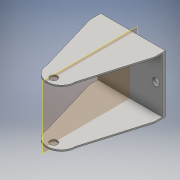
# Autodesk Inventor part: Thin Wheel Mount
Saved by Autodesk Inventor 2016 (Build 200138000, 138)
## iProperties
Created: 2016-05-08
Part Number: Thin Wheel Mount
Material: Generic
Document SubType Name: Modeling
Designer: Kenneth Daniel
Density: 1 g/cm^3
Appearance: Default
Author: Kenneth Daniel
Autodesk Inventor part; units mm, degrees
ref_plane "YZ Plane" through (0, 0, 0) normal (1, 0, 0) x (0, 1, 0)
ref_plane "XZ Plane" through (0, 0, 0) normal (0, 1, 0) x (-1, 0, 0)
ref_plane "XY Plane" through (0, 0, 0) normal (0, 0, 1) x (1, 0, 0)
sketch "Sketch1" plane through (0, 0, 0) normal (0, 0, 1) x (1, 0, 0)
  line L0 (-22.5, -30) -> (-22.5, 30)
  line L1 (-22.5, 30) -> (22.5, 30)
  line L2 (22.5, 30) -> (22.5, -30)
  line L3 (22.5, -30) -> (-22.5, -30)
  line L4 (-22.5, -30) -> (22.5, 30) construction
  line L5 (-22.5, 30) -> (22.5, -30) construction
  line L6 (-22.5, 30) -> (-22.5, 22.5)
  line L7 (0, -30) -> (0, -20)
  line L8 (0, -20) -> (-10, -20)
  line L9 (-10, -20) -> (10, -20)
  line L10 (-22.5, 22.5) -> (-10, -20)
  line L11 (22.5, 30) -> (22.5, 22.5)
  line L12 (22.5, 22.5) -> (10, -20)
  arc A0 (-10, -20) -> (10, -20) centre (0, -20) ccw
  point P0 (0, 0)
  dimension "d0" = 60
  dimension "d1" = 45
  dimension "d2" = 7.5
  dimension "d3" = 10
  dimension "d4" = 10
  dimension "d5" = 20
  dimension "d6" = 7.5
  constraints: 26 end point, 3 midpoint, 3 point on circle, 3 point on line, 2 parallel, 2 perpendicular, 2 vertical, 1 centre point
  measures "d0" distance of L0.start L0.end
  measures "d1" distance of L0.end L1.end
  measures "d2" distance of L0.end L6.end
  measures "d3" distance of L7.start L7.end
  measures "d4" distance of L7.end L8.end
  measures "d5" distance of L8.end L9.end
  measures "d6" distance of L1.end L11.end
extrude "Extrusion1" add sketch "Sketch1" along normal blind 40 contours L0 L1 L2 L12 L9 L8 L10 | A0 L8 L7 | L7 L9 A0
sketch "Sketch2" plane through (0, 0, 0) normal (1, 0, 0) x (0, 1, 0)
  line L0 (30, 0) -> (30, 40) projected
  line L1 (30, 40) -> (30, 0)
  line L2 (-20, 0) -> (-30, 0) projected
  line L3 (30, 0) -> (-30, 0)
  line L4 (-30, 0) -> (-30, 1)
  line L5 (-30, 0) -> (-30, 40) projected
  line L6 (30, 40) -> (-30, 40)
  line L7 (-30, 40) -> (-30, 39)
  line L8 (-30, 39) -> (27.8612, 39)
  line L9 (30, 40) -> (22.5, 40) projected
  line L10 (-30, 1) -> (27.8612, 1)
  line L11 (27.8612, 1) -> (27.8612, 39)
  line L12 (-30, 39) -> (-30, 1)
  point P0 (0, 0)
  dimension "d9" = 1
  dimension "d10" = 1
  constraints: 18 end point, 2 horizontal, 2 perpendicular, 2 point on line, 1 collinear, 1 parallel, 1 vertical
  measures "d9" distance of L2.end L4.end
  measures "d10" distance of L5.end L7.end
extrude "Extrusion2" cut sketch "Sketch2" along normal through all both and the other way through all contours L5 L8 L11 L10
sketch "Sketch3" plane through (0, 0, 40) normal (0, 0, 1) x (1, 0, 0)
  arc A0 (-10, -20) -> (10, -20) centre (0, -20) ccw projected
  line L0 (10, -20) -> (22.5, 22.5) projected
  line L1 (22.5, 22.5) -> (22.5, 30) projected
  line L2 (22.5, 30) -> (-22.5, 30) projected
  line L3 (-22.5, 30) -> (-22.5, 22.5) projected
  line L4 (-22.5, 22.5) -> (-10, -20) projected
  circle A1 centre (0, -25.2901) radius 2.5
  point P0 (0, 0)
  dimension "d13" = 5
  constraints: 1 centre point
  measures "d13" diameter of A1
extrude "Extrusion3" cut sketch "Sketch3" against normal blind 40 contours A1
sketch "Sketch4" plane through (-22.5, 30, 0) normal (0, 1, 0) x (1, 0, 0)
  line L0 (45, -40) -> (0, -40) projected
  line L1 (45, 0) -> (0, 0) projected
  line L2 (0, -40) -> (45, 0) construction
  line L3 (0, 0) -> (0, -40) projected
  line L4 (0, 0) -> (45, -40) construction
  line L5 (0, -20) -> (45, -20) construction
  circle A0 centre (4.5627, -20) radius 2.5
  point P0 (22.5, 0)
  dimension "d16" = 5
  constraints: 6 end point, 1 centre point, 1 horizontal, 1 midpoint, 1 point on line
  measures "d16" diameter of A0
extrude "Extrusion4" cut sketch "Sketch4" against normal blind 10
ref_plane "Work Plane1" through (0, 22.5, 0) normal (1, 0, 0) x (0, 0, -1)
mirror "Mirror1" about plane through (0, 22.5, 0) normal (1, 0, 0) of "Extrusion4"
body "Solid1"
